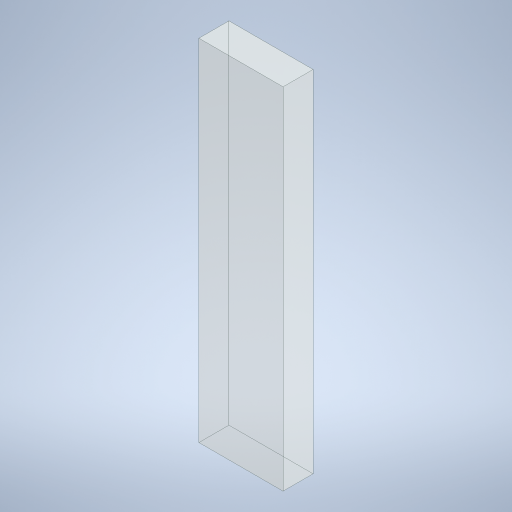
# Autodesk Inventor part: 玻璃門
Saved by Autodesk Inventor 2024.2 (Build 282272000, 272)
## iProperties
Created: 2024-06-05
Part Number: 玻璃門
Material: 玻璃
Document SubType Name: Modeling
Designer: User
Density: 2.18 g/cm^3
Appearance: 明亮
Author: User
Autodesk Inventor part; units mm, degrees
ref_plane "YZ Plane" through (0, 0, 0) normal (1, 0, 0) x (0, 1, 0)
ref_plane "XZ Plane" through (0, 0, 0) normal (0, 1, 0) x (-1, 0, 0)
ref_plane "XY Plane" through (0, 0, 0) normal (0, 0, 1) x (1, 0, 0)
sketch "草圖1" plane through (0, 0, 0) normal (0, 0, 1) x (1, 0, 0)
  line L0 (0, 0) -> (1.4, 0)
  line L1 (1.4, 0) -> (1.4, -5.825)
  line L2 (1.4, -5.825) -> (0, -5.825)
  line L3 (0, -5.825) -> (0, 0)
  dimension "d0" = 1.4
  dimension "d1" = 5.825
  constraints: 8 end point, 2 parallel, 1 horizontal, 1 perpendicular
  measures "d0" distance of L0.start L0.end
  measures "d1" distance of L0.end L1.end
extrude "擠出1" add sketch "草圖1" along normal blind 0.5
